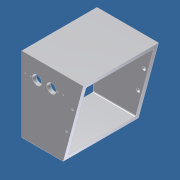
# Autodesk Inventor part: GE-12059
Saved by Autodesk Inventor 2012 (Build 160160000, 160)
## iProperties
Created: 2011-07-19
Part Number: GE-12059
Document SubType Name: Modeling
Designer: mcyr
Density: 1 g/cm^3
Description: Sensor Box
Material: Default
Title: Sensor Box
Author: mcyr
Autodesk Inventor part; units mm, degrees
ref_plane "YZ Plane" through (0, 0, 0) normal (1, 0, 0) x (0, 1, 0)
ref_plane "XZ Plane" through (0, 0, 0) normal (0, 1, 0) x (-1, 0, 0)
ref_plane "XY Plane" through (0, 0, 0) normal (0, 0, 1) x (1, 0, 0)
sketch "Sketch1" plane through (0, 0, 0) normal (0, 0, 1) x (1, 0, 0)
  line L0 (0, 0) -> (0, 254)
  line L1 (0, 254) -> (207.7591, 254)
  line L2 (207.7591, 254) -> (139.7, 0)
  line L3 (139.7, 0) -> (0, 0)
  dimension "d0" = 254
  dimension "d2" = 139.7
  dimension "d24" = 75
  constraints: 8 end point, 1 parallel, 1 perpendicular, 1 vertical
  measures "d0" distance of L0.start L0.end
  measures "d2" distance of L2.end L0.start
  measures "d24" angle of L1 L2
extrude "Extrusion1" add sketch "Sketch1" along normal blind 254
sketch "Sketch2" plane through (0, 0, 0) normal (-1, 0, 0) x (0, 0, 1)
  line L0 (254, 0) -> (254, 254) projected
  line L1 (0, 254) -> (254, 254) projected
  line L2 (0, 0) -> (0, 254) projected
  line L3 (0, 0) -> (254, 0) projected
  line L4 (241.3, 241.3) -> (241.3, 12.7)
  line L5 (241.3, 12.7) -> (12.7, 12.7)
  line L6 (12.7, 12.7) -> (12.7, 241.3)
  line L7 (12.7, 241.3) -> (241.3, 241.3)
  dimension "d5" = 12.7
  constraints: 8 end point, 3 other
  measures "d5" distance between parallel lines of L1 L7
extrude "Extrusion2" cut sketch "Sketch2" against normal blind 209.55 contours L4 L5 L6 L7
sketch "Sketch6" plane through (0, 12.7, 241.3) normal (0, 0, -1) x (-1, 0, 0)
  line L0 (-143.103, 0) -> (-204.3561, 228.6) projected
  line L1 (0, 241.3) -> (-207.7591, 241.3) projected
  line L2 (-207.7591, 241.3) -> (-191.6487, 245.6168)
  point P0 (0, -12.7)
  point P1 (-139.7, -12.7)
  point P2 (-171.2502, 154.116)
  point P3 (-151.5282, 80.5124)
  point P4 (-203.2, 224.2852)
  dimension "d73" = 93.6625
  dimension "d74" = 169.8625
  dimension "d75" = 12.7
  dimension "d76" = 12.7
  constraints: 2 end point, 1 perpendicular
  measures "d73" distance from line of point (-171.25, 154.116) L2
  measures "d74" distance from line of point (-151.528, 80.512) L2
  measures "d75" distance from line of point (-171.25, 154.116) L0
  measures "d76" distance from line of point (-151.528, 80.512) L0
sketch "Sketch7" plane through (0, 12.7, 12.7) normal (0, 0, 1) x (1, 0, 0)
  point P0 (0, -12.7)
  point P1 (171.2502, 154.116)
  point P2 (151.5282, 80.5124)
hole "Hole1" at (51.435, 193.675, 254) direction (0, 0, -1) diameter 31.75 end through all
hole "Hole2" at (171.2502, 166.816, 12.7) direction (0, 0, -1) diameter 6.35 depth 25.4 tip angle 118 countersink diameter 12.7 countersink angle 82
hole "Hole3" at (151.5282, 93.2124, 12.7) direction (0, 0, -1) diameter 6.35 depth 25.4 tip angle 118 countersink diameter 12.7 countersink angle 82
hole "Hole4" at (171.2502, 166.816, 241.3) direction (0, 0, 1) diameter 6.35 depth 25.4 tip angle 118 countersink diameter 12.7 countersink angle 82
hole "Hole5" at (151.5282, 93.2124, 241.3) direction (0, 0, 1) diameter 6.35 depth 25.4 tip angle 118 countersink diameter 12.7 countersink angle 82
fillet "Fillet1" radius 3.175 4 edges at (102.1781, 241.3, 12.7) (102.1781, 241.3, 241.3) (71.5515, 12.7, 241.3) (71.5515, 12.7, 12.7)
pattern_linear "Rectangular Pattern2" count 2 spacing 48.895 along (1, 0, 0) of "Hole1"
hole "Hole6" at (29.4894, 193.675, 254) direction (0, 0, -1) diameter 3.683 end through all thread size "10-24 UNC" class "2B" standard "ANSI Unified Screw Threads"
pattern_linear "Rectangular Pattern3" count 2 spacing 17.78 along (-1, 0, 0) of "Hole6"
pattern_linear "Rectangular Pattern4" count 2 spacing 110.49 along (1, 0, 0) of "Hole6", "Rectangular Pattern3"
equation "\"d76\" = d75"
body "Solid1"
